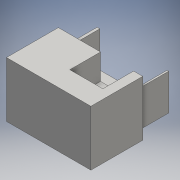
# Autodesk Inventor part: 240503_3Dsketch02
Saved by Autodesk Inventor 2016 (Build 200138000, 138)
## iProperties
Created: 2024-05-03
Part Number: 240503_3Dsketch02
Material: 일반
Document SubType Name: Modeling
Designer: pc
Density: 1 g/cm^3
Appearance: 기본값
Author: pc
Autodesk Inventor part; units mm, degrees
ref_plane "YZ Plane" through (0, 0, 0) normal (1, 0, 0) x (0, 1, 0)
ref_plane "XZ Plane" through (0, 0, 0) normal (0, 1, 0) x (-1, 0, 0)
ref_plane "XY Plane" through (0, 0, 0) normal (0, 0, 1) x (1, 0, 0)
sketch "스케치1" plane through (0, 0, 0) normal (0, 0, 1) x (1, 0, 0)
  line L0 (68.5732, -42.1218) -> (-68.5732, -42.1218)
  line L1 (-68.5732, -42.1218) -> (-68.5732, 42.1218)
  line L2 (-68.5732, 42.1218) -> (68.5732, 42.1218)
  line L3 (68.5732, 42.1218) -> (68.5732, -42.1218)
  line L4 (68.5732, -42.1218) -> (-68.5732, 42.1218) construction
  line L5 (-68.5732, -42.1218) -> (68.5732, 42.1218) construction
  point P0 (0, 0)
  constraints: 12 end point, 2 midpoint, 2 parallel, 1 horizontal, 1 perpendicular
extrude "돌출1" add sketch "스케치1" along normal blind 90
sketch "스케치2" plane through (-68.5732, 42.1218, 0) normal (0, 1, 0) x (1, 0, 0)
  line L0 (0, -90) -> (137.1464, -90) projected
  line L1 (68.5732, -90) -> (122.3358, -90)
  line L2 (122.3358, -90) -> (122.3358, -48.4921)
  line L3 (122.3358, -48.4921) -> (68.5732, -48.4921)
  line L4 (68.5732, -48.4921) -> (68.5732, -90)
  point P0 (68.5732, 0)
  constraints: 8 end point, 2 parallel, 1 horizontal, 1 midpoint, 1 perpendicular
extrude "돌출2" cut sketch "스케치2" against normal blind 50
sketch "스케치3" plane through (-68.5732, 42.1218, 0) normal (0, 1, 0) x (1, 0, 0)
  line L0 (13.0375, -71.9969) -> (13.0375, -9.4777)
  line L1 (13.0375, -9.4777) -> (129.4297, -9.4777)
  line L2 (129.4297, -9.4777) -> (129.4297, -68.3389)
  line L3 (129.4297, -68.3389) -> (126.7693, -68.3389)
  line L4 (126.7693, -68.3389) -> (126.7693, -13.8008)
  line L5 (126.7693, -13.8008) -> (17.3606, -13.8008)
  line L6 (17.3606, -13.8008) -> (17.3606, -71.9969)
  line L7 (17.3606, -71.9969) -> (13.0375, -71.9969)
  point P0 (68.5732, 0)
  constraints: 16 end point, 7 perpendicular, 1 vertical
extrude "돌출3" add sketch "스케치3" along normal blind 50
